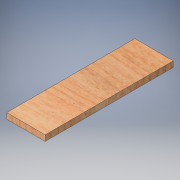
# Autodesk Inventor part: Base
Saved by Autodesk Inventor 2016 SP2 (Build 200236200, 236)
## iProperties
Created: 2017-06-01
Part Number: Base
Material: Abedul
Document SubType Name: Modeling
Designer: ssant
Density: 0.512 g/cm^3
Appearance: Abedul - Natural brillo medio
Author: ssant
Autodesk Inventor part; units mm, degrees
ref_plane "YZ Plane" through (0, 0, 0) normal (1, 0, 0) x (0, 1, 0)
ref_plane "XZ Plane" through (0, 0, 0) normal (0, 1, 0) x (-1, 0, 0)
ref_plane "XY Plane" through (0, 0, 0) normal (0, 0, 1) x (1, 0, 0)
sketch "Boceto1" plane through (0, 0, 0) normal (0, 1, 0) x (-1, 0, 0)
  line L0 (30, 100) -> (-30, 100)
  line L1 (-30, 100) -> (-30, -100)
  line L2 (-30, -100) -> (30, -100)
  line L3 (30, -100) -> (30, 100)
  point P0 (0, 0)
  point P1 (30, 0)
  point P2 (0, 100)
  dimension "d0" = 60
  dimension "d1" = 200
  constraints: 8 end point, 2 midpoint, 2 parallel, 1 horizontal, 1 horizontal alignment, 1 perpendicular, 1 vertical alignment
  measures "d0" distance of L2.end L1.end
  measures "d1" distance of L1.end L0.end
extrude "Extrusión1" add sketch "Boceto1" along normal blind 9
